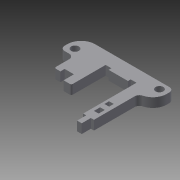
# Autodesk Inventor part: Gripper V 10.1 servo bracket bottom 6mm
Saved by Autodesk Inventor 2015 (Build 190159000, 159)
## iProperties
Created: 2015-06-23
Part Number: Gripper V 10.1 servo bracket bottom 6mm
Material: Generic
Document SubType Name: Modeling
Designer: Stackpole
Density: 1 g/cm^3
Appearance: Default
Author: Stackpole
Autodesk Inventor part; units mm, degrees
ref_plane "YZ Plane" through (0, 0, 0) normal (1, 0, 0) x (0, 1, 0)
ref_plane "XZ Plane" through (0, 0, 0) normal (0, 1, 0) x (-1, 0, 0)
ref_plane "XY Plane" through (0, 0, 0) normal (0, 0, 1) x (1, 0, 0)
sketch "Sketch1" plane through (0, 0, 0) normal (0, 0, 1) x (1, 0, 0)
  line L0 (0, 4.25) -> (0, 7)
  line L1 (0, 7) -> (6, 7)
  line L2 (6, 7) -> (6, 0.3)
  line L3 (6, 0.3) -> (11, 0.3)
  line L4 (11, 0.3) -> (11, 22.5)
  line L5 (-4, 4.25) -> (0, 4.25)
  line L6 (30.939, 22.5) -> (27.2275, 22.5)
  line L7 (27.2275, 22.5) -> (27.2275, 20.708)
  line L8 (27.2275, 20.708) -> (14.7135, 20.708)
  line L9 (14.7135, 20.708) -> (14.7135, 22.5)
  line L10 (14.7135, 22.5) -> (11, 22.5)
  line L11 (30.939, 22.5) -> (30.939, -12)
  line L12 (30.939, -12) -> (32.939, -12)
  line L13 (32.939, -12) -> (32.939, -17.9)
  line L14 (32.939, -17.9) -> (35.939, -17.9)
  line L15 (35.939, -17.9) -> (35.939, -12)
  line L16 (35.939, -12) -> (37.939, -12)
  line L17 (37.939, -12) -> (37.939, 17)
  line L18 (37.939, 17) -> (46.9695, 17)
  line L19 (46.9695, 17) -> (46.9695, 30.708)
  line L20 (-4, 4.25) -> (-4, 17)
  line L21 (-4, 17) -> (-13.0305, 17)
  line L22 (-13.0305, 17) -> (-13.0305, 30.708)
  line L23 (46.9695, 30.708) -> (-13.0305, 30.708)
  dimension "d0" = 6
  dimension "d1" = 6.7
  dimension "d3" = 5
  dimension "d10" = 4
  dimension "d12" = 2.75
  dimension "d15" = 1.792
  dimension "d20" = 3
  dimension "d21" = 2
  dimension "d22" = 5.9
  dimension "d23" = 12.514
  dimension "d24" = 19.939
  dimension "d25" = 3.7135
  dimension "d42" = 13.708
  dimension "d43" = 19
  dimension "d48" = 7
  dimension "d50" = 60
  dimension "d51" = 41.939
  dimension "d52" = 9.0305
  dimension "d65" = 10
  dimension "d66" = 29
  constraints: 48 end point, 17 perpendicular, 4 vertical, 3 horizontal, 2 point on line, 1 collinear
  measures "d0" distance of L0.end L1.end
  measures "d1" distance of L1.end L2.end
  measures "d3" distance of L2.end L3.end
  measures "d10" distance of L5.start L0.start
  measures "d12" distance of L0.start L0.end
  measures "d15" distance of L6.end L7.end
  measures "d20" distance of L13.end L14.end
  measures "d21" distance of L11.end L12.end
  measures "d22" distance of L14.end L15.end
  measures "d23" distance of L7.end L8.end
  measures "d24" distance between parallel lines of L11 L4
  measures "d25" distance of L9.end L4.end
  measures "d42" distance between parallel lines of L1 L8
  measures "d43" distance between parallel lines of L1 L12
  measures "d48" distance between parallel lines of L17 L11
  measures "d50" distance of L19.end L22.end
  measures "d51" distance between parallel lines of L20 L17
  measures "d52" distance of L17.end L18.end
  measures "d65" distance between parallel lines of L23 L8
  measures "d66" distance between parallel lines of L16 L18
extrude "Extrusion1" add sketch "Sketch1" along normal blind 6
sketch "Sketch2" plane through (0, 0, 6) normal (0, 0, 1) x (1, 0, 0)
  line L0 (35.45, 0.264) -> (32.45, 0.264)
  line L1 (32.45, 0.264) -> (32.45, 3.264)
  line L2 (32.45, 3.264) -> (35.45, 3.264)
  line L3 (35.45, 3.264) -> (35.45, 0.264)
  line L4 (34.939, 35.708) -> (-1, 35.708) projected
  line L5 (30.939, 22.5) -> (30.939, -12) projected
  line L6 (32.939, -17.9) -> (35.939, -17.9) projected
  point P0 (0, 0)
  dimension "d26" = 3
  dimension "d27" = 3
  dimension "d61" = 18.164
  dimension "d62" = 1.511
  constraints: 8 end point, 2 parallel, 1 horizontal, 1 perpendicular
  measures "d26" distance of L0.end L1.end
  measures "d27" distance of L0.start L0.end
  measures "d61" distance between parallel lines of L6 L0
  measures "d62" distance between parallel lines of L5 L1
extrude "Extrusion2" cut sketch "Sketch2" against normal blind 10
sketch "Sketch3" plane through (0, 0, 0) normal (0, 0, -1) x (-1, 0, 0)
  line L0 (-32.939, -7) -> (-35.939, -7)
  line L1 (-35.939, -7) -> (-35.939, -3)
  line L2 (-35.939, -3) -> (-32.939, -3)
  line L3 (-32.939, -3) -> (-32.939, -7)
  line L4 (-35.939, -12) -> (-37.939, -12) projected
  line L5 (-37.939, -12) -> (-37.939, 17) projected
  point P0 (0, 0)
  dimension "d32" = 3
  dimension "d33" = 4
  dimension "d34" = 5
  dimension "d63" = 2
  constraints: 8 end point, 2 parallel, 1 horizontal, 1 perpendicular
  measures "d32" distance of L1.end L2.end
  measures "d33" distance of L0.end L1.end
  measures "d34" distance between parallel lines of L4 L0
  measures "d63" distance between parallel lines of L5 L1
extrude "Extrusion3" cut sketch "Sketch3" against normal blind 10
fillet "Fillet4" radius 1 2 edges at (11, 0.3, 3) (-4, 4.25, 3)
sketch "Sketch4" plane through (0, 0, 6) normal (0, 0, 1) x (1, 0, 0)
  circle A0 centre (41.9595, 26.3) radius 2.5
  circle A1 centre (-8.0305, 21.7) radius 2.5
  line L0 (-13.0305, 30.708) -> (-13.0305, 17) projected
  line L1 (-13.0305, 17) -> (-4, 17) projected
  line L2 (46.9695, 17) -> (46.9695, 30.708) projected
  line L3 (37.939, 17) -> (46.9695, 17) projected
  point P0 (0, 0)
  dimension "d45" = 5
  dimension "d46" = 5
  dimension "d53" = 5
  dimension "d67" = 4.7
  dimension "d70" = 5.01
  dimension "d71" = 9.3
  constraints: 2 centre point
  measures "d45" diameter of A0
  measures "d46" diameter of A1
  measures "d53" distance from line of L0 A1.centre
  measures "d67" distance from line of L1 A1.centre
  measures "d70" distance from line of L2 A0.centre
  measures "d71" distance from line of L3 A0.centre
extrude "Extrusion4" cut sketch "Sketch4" against normal blind 10
fillet "Fillet6" radius 9 2 edges at (-13.0305, 30.708, 3) (46.9695, 17, 3)
fillet "Fillet7" radius 3 4 edges at (37.939, 17, 3) (46.9695, 30.708, 3) (-4, 17, 3) (-13.0305, 17, 3)
body "Solid1"
